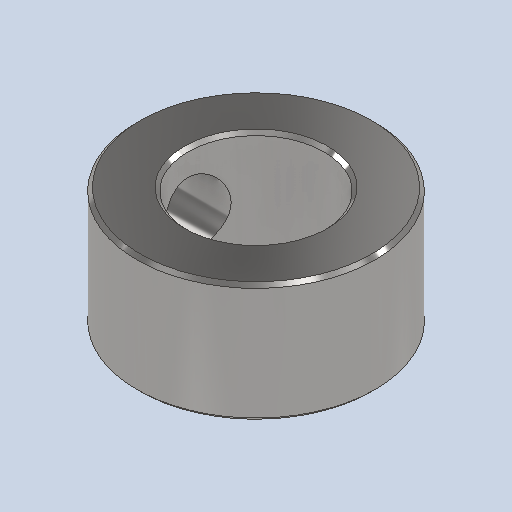
# Autodesk Inventor part: 8mmShaftCollar
Saved by Autodesk Inventor 2024 (Build 280153000, 153)
## iProperties
Created: 2021-11-12
Part Number: 8mmShaftCollar
Material: Generic
Document SubType Name: Modeling
Designer: Henry Cawley
Density: 1 g/cm^3
Appearance: Steel - Polished
Author: Henry Cawley
Autodesk Inventor part; units mm, degrees
ref_plane "YZ Plane" through (0, 0, 0) normal (1, 0, 0) x (0, 1, 0)
ref_plane "XZ Plane" through (0, 0, 0) normal (0, 1, 0) x (-1, 0, 0)
ref_plane "XY Plane" through (0, 0, 0) normal (0, 0, 1) x (1, 0, 0)
sketch "Sketch1" plane through (0, 0, 0) normal (0, 1, 0) x (-1, 0, 0)
  circle A0 centre (0, 0) radius 7
  circle A1 centre (0, 0) radius 4
  dimension "d0" = 14
  dimension "d1" = 8
  constraints: 2 centre point, 2 coincident
  measures "d0" diameter of A0
  measures "d1" diameter of A1
extrude "Extrusion1" add sketch "Sketch1" along normal blind 7
chamfer "Chamfer1" distance 0.2 angle 45 4 edges at (7, 7, 0) (4, 7, 0) (7, 0, 0) (4, 0, 0)
sketch "Sketch2" plane through (0, 0, 0) normal (0, 1, 0) x (-1, 0, 0)
  point P0 (0, 0)
sketch "Sketch3" plane through (0, 0, 0) normal (1, 0, 0) x (0, 1, 0)
  circle A0 centre (3.5, 0) radius 2
  line L0 (7, -4.2) -> (7, 4.2) projected
  point P0 (0, 0)
  dimension "d7" = 4
  dimension "d8" = 3.5
  constraints: 1 centre point
  measures "d7" diameter of A0
  measures "d8" distance from line of L0 A0.centre
extrude "Extrusion2" cut sketch "Sketch3" against normal blind 7
body "Solid1"
